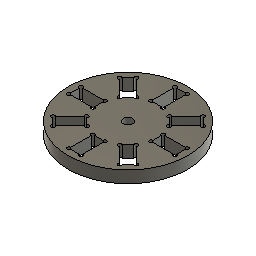
Yatsı Mıknatıs Tutucu v15 (Autodesk Fusion 360 design; units mm, degrees)
Autodesk Fusion 360 part; units mm, degrees
sketch "Eskiz1" plane through (0, 0, 0) normal (0, 1, 0) x (1, 0, 0)
  circle A0 centre (0, 0) radius 20
  circle A1 centre (0, 0) radius 50
  line L0 (-5, 44.3809) -> (5, 44.3809)
  line L1 (5, 44.3809) -> (5, 24.3809)
  line L2 (5, 24.3809) -> (-5, 24.3809)
  line L3 (-5, 24.3809) -> (-5, 44.3809)
  circle A2 centre (-5, 24.3809) radius 1.5
  circle A3 centre (5, 24.3809) radius 1.5
  circle A4 centre (-5, 44.3809) radius 1.5
  circle A5 centre (5, 44.3809) radius 1.5
  circle A6 centre (-34.9176, 27.8465) radius 1.5
  line L4 (-34.9176, 27.8465) -> (-27.8465, 34.9176)
  line L5 (-20.7754, 13.7044) -> (-34.9176, 27.8465)
  line L6 (-13.7044, 20.7754) -> (-20.7754, 13.7044)
  line L7 (-27.8465, 34.9176) -> (-13.7044, 20.7754)
  circle A7 centre (-27.8465, 34.9176) radius 1.5
  circle A8 centre (-20.7754, 13.7044) radius 1.5
  circle A9 centre (-13.7044, 20.7754) radius 1.5
  circle A10 centre (-44.3809, -5) radius 1.5
  line L8 (-44.3809, -5) -> (-44.3809, 5)
  line L9 (-24.3809, -5) -> (-44.3809, -5)
  line L10 (-24.3809, 5) -> (-24.3809, -5)
  line L11 (-44.3809, 5) -> (-24.3809, 5)
  circle A11 centre (-44.3809, 5) radius 1.5
  circle A12 centre (-24.3809, -5) radius 1.5
  circle A13 centre (-24.3809, 5) radius 1.5
  circle A14 centre (-27.8465, -34.9176) radius 1.5
  line L12 (-27.8465, -34.9176) -> (-34.9176, -27.8465)
  line L13 (-13.7044, -20.7754) -> (-27.8465, -34.9176)
  line L14 (-20.7754, -13.7044) -> (-13.7044, -20.7754)
  line L15 (-34.9176, -27.8465) -> (-20.7754, -13.7044)
  circle A15 centre (-34.9176, -27.8465) radius 1.5
  circle A16 centre (-13.7044, -20.7754) radius 1.5
  circle A17 centre (-20.7754, -13.7044) radius 1.5
  circle A18 centre (5, -44.3809) radius 1.5
  line L16 (5, -44.3809) -> (-5, -44.3809)
  line L17 (5, -24.3809) -> (5, -44.3809)
  line L18 (-5, -24.3809) -> (5, -24.3809)
  line L19 (-5, -44.3809) -> (-5, -24.3809)
  circle A19 centre (-5, -44.3809) radius 1.5
  circle A20 centre (5, -24.3809) radius 1.5
  circle A21 centre (-5, -24.3809) radius 1.5
  circle A22 centre (34.9176, -27.8465) radius 1.5
  line L20 (34.9176, -27.8465) -> (27.8465, -34.9176)
  line L21 (20.7754, -13.7044) -> (34.9176, -27.8465)
  line L22 (13.7044, -20.7754) -> (20.7754, -13.7044)
  line L23 (27.8465, -34.9176) -> (13.7044, -20.7754)
  circle A23 centre (27.8465, -34.9176) radius 1.5
  circle A24 centre (20.7754, -13.7044) radius 1.5
  circle A25 centre (13.7044, -20.7754) radius 1.5
  circle A26 centre (44.3809, 5) radius 1.5
  line L24 (44.3809, 5) -> (44.3809, -5)
  line L25 (24.3809, 5) -> (44.3809, 5)
  line L26 (24.3809, -5) -> (24.3809, 5)
  line L27 (44.3809, -5) -> (24.3809, -5)
  circle A27 centre (44.3809, -5) radius 1.5
  circle A28 centre (24.3809, 5) radius 1.5
  circle A29 centre (24.3809, -5) radius 1.5
  circle A30 centre (27.8465, 34.9176) radius 1.5
  line L28 (27.8465, 34.9176) -> (34.9176, 27.8465)
  line L29 (13.7044, 20.7754) -> (27.8465, 34.9176)
  line L30 (20.7754, 13.7044) -> (13.7044, 20.7754)
  line L31 (34.9176, 27.8465) -> (20.7754, 13.7044)
  circle A31 centre (34.9176, 27.8465) radius 1.5
  circle A32 centre (13.7044, 20.7754) radius 1.5
  circle A33 centre (20.7754, 13.7044) radius 1.5
  circle A34 centre (0, 0) radius 3.9
  point P0 (-5, 0)
  point P1 (5, 0)
  dimension "d1" = 40
  dimension "d2" = 100
  dimension "d3" = 5
  dimension "d4" = 5
  dimension "d5" = 10
  dimension "d6" = 20
  dimension "d9" = 44.3809
  dimension "d10" = 3
  dimension "d11" = 3
  dimension "d12" = 3
  dimension "d13" = 3
  dimension "d15" = 360
  dimension "d16" = 7.8
  constraint coincident A0.centre A1.centre
  constraint concentric A0 A1
  constraint horizontal L0
  constraint vertical L1
  constraint horizontal L2
  constraint vertical L3
  constraint coincident L2.end L3.start
  constraint coincident L1.end L2.start
  constraint coincident L0.start L3.end
  constraint coincident L0.end L1.start
  measures "d1" diameter of A0
  measures "d2" diameter of A1
  measures "d3" distance of A0.centre P0
  measures "d4" distance of A0.centre P1
  measures "d5" distance of L0.start L0.end
  measures "d6" distance of L0.start L2.end
  measures "d9" distance of P0 L0.start
  measures "d10" diameter of A2
  measures "d11" diameter of A3
  measures "d12" diameter of A4
  measures "d13" diameter of A5
  measures "d16" diameter of A34
extrude "Ekstrüde Et1" add sketch "Eskiz1" along normal blind 10 contours A0 | A1
extrude "Ekstrüde Et2" add sketch "Eskiz1" along normal blind 6.5 contours A0
sketch "Eskiz2" plane through (0, 10, 0) normal (0, 1, 0) x (-1, 0, 0)
  arc A0 (-14.765, -21.8361) -> (-14.765, -19.7148) centre (-13.7044, -20.7754) ccw
  line L0 (-14.765, -21.8361) -> (-26.7858, -33.8569)
  arc A1 (-28.9072, -33.8569) -> (-26.7858, -33.8569) centre (-27.8465, -34.9176) ccw
  line L1 (-28.9072, -33.8569) -> (-33.8569, -28.9072)
  arc A2 (-33.8569, -26.7858) -> (-33.8569, -28.9072) centre (-34.9176, -27.8465) ccw
  line L2 (-33.8569, -26.7858) -> (-21.8361, -14.765)
  arc A3 (-19.7148, -14.765) -> (-21.8361, -14.765) centre (-20.7754, -13.7044) ccw
  line L3 (-19.7148, -14.765) -> (-14.765, -19.7148)
  circle A4 centre (0, 0) radius 3.9
  arc A5 (-3.5, -24.3809) -> (-5, -25.8809) centre (-5, -24.3809) ccw
  line L4 (-3.5, -24.3809) -> (3.5, -24.3809)
  arc A6 (5, -25.8809) -> (3.5, -24.3809) centre (5, -24.3809) ccw
  line L5 (5, -25.8809) -> (5, -42.8809)
  arc A7 (3.5, -44.3809) -> (5, -42.8809) centre (5, -44.3809) ccw
  line L6 (3.5, -44.3809) -> (-3.5, -44.3809)
  arc A8 (-5, -42.8809) -> (-3.5, -44.3809) centre (-5, -44.3809) ccw
  line L7 (-5, -42.8809) -> (-5, -25.8809)
  arc A9 (21.8361, -14.765) -> (19.7148, -14.765) centre (20.7754, -13.7044) ccw
  line L8 (21.8361, -14.765) -> (33.8569, -26.7858)
  arc A10 (33.8569, -28.9072) -> (33.8569, -26.7858) centre (34.9176, -27.8465) ccw
  line L9 (33.8569, -28.9072) -> (28.9072, -33.8569)
  arc A11 (26.7858, -33.8569) -> (28.9072, -33.8569) centre (27.8465, -34.9176) ccw
  line L10 (26.7858, -33.8569) -> (14.765, -21.8361)
  arc A12 (14.765, -19.7148) -> (14.765, -21.8361) centre (13.7044, -20.7754) ccw
  line L11 (14.765, -19.7148) -> (19.7148, -14.765)
  arc A13 (25.8809, 5) -> (24.3809, 3.5) centre (24.3809, 5) ccw
  line L12 (25.8809, 5) -> (42.8809, 5)
  arc A14 (44.3809, 3.5) -> (42.8809, 5) centre (44.3809, 5) ccw
  line L13 (44.3809, 3.5) -> (44.3809, -3.5)
  arc A15 (42.8809, -5) -> (44.3809, -3.5) centre (44.3809, -5) ccw
  line L14 (42.8809, -5) -> (25.8809, -5)
  arc A16 (24.3809, -3.5) -> (25.8809, -5) centre (24.3809, -5) ccw
  line L15 (24.3809, -3.5) -> (24.3809, 3.5)
  arc A17 (14.765, 21.8361) -> (14.765, 19.7148) centre (13.7044, 20.7754) ccw
  line L16 (14.765, 21.8361) -> (26.7858, 33.8569)
  arc A18 (28.9072, 33.8569) -> (26.7858, 33.8569) centre (27.8465, 34.9176) ccw
  line L17 (28.9072, 33.8569) -> (33.8569, 28.9072)
  arc A19 (33.8569, 26.7858) -> (33.8569, 28.9072) centre (34.9176, 27.8465) ccw
  line L18 (33.8569, 26.7858) -> (21.8361, 14.765)
  arc A20 (19.7148, 14.765) -> (21.8361, 14.765) centre (20.7754, 13.7044) ccw
  line L19 (19.7148, 14.765) -> (14.765, 19.7148)
  arc A21 (-5, 25.8809) -> (-3.5, 24.3809) centre (-5, 24.3809) ccw
  line L20 (-5, 25.8809) -> (-5, 42.8809)
  arc A22 (-3.5, 44.3809) -> (-5, 42.8809) centre (-5, 44.3809) ccw
  line L21 (-3.5, 44.3809) -> (3.5, 44.3809)
  arc A23 (5, 42.8809) -> (3.5, 44.3809) centre (5, 44.3809) ccw
  line L22 (5, 42.8809) -> (5, 25.8809)
  arc A24 (3.5, 24.3809) -> (5, 25.8809) centre (5, 24.3809) ccw
  line L23 (3.5, 24.3809) -> (-3.5, 24.3809)
  arc A25 (-33.8569, 28.9072) -> (-33.8569, 26.7858) centre (-34.9176, 27.8465) ccw
  line L24 (-33.8569, 28.9072) -> (-28.9072, 33.8569)
  arc A26 (-26.7858, 33.8569) -> (-28.9072, 33.8569) centre (-27.8465, 34.9176) ccw
  line L25 (-26.7858, 33.8569) -> (-14.765, 21.8361)
  arc A27 (-14.765, 19.7148) -> (-14.765, 21.8361) centre (-13.7044, 20.7754) ccw
  line L26 (-14.765, 19.7148) -> (-19.7148, 14.765)
  arc A28 (-21.8361, 14.765) -> (-19.7148, 14.765) centre (-20.7754, 13.7044) ccw
  line L27 (-21.8361, 14.765) -> (-33.8569, 26.7858)
  arc A29 (-44.3809, -3.5) -> (-42.8809, -5) centre (-44.3809, -5) ccw
  line L28 (-44.3809, -3.5) -> (-44.3809, 3.5)
  arc A30 (-42.8809, 5) -> (-44.3809, 3.5) centre (-44.3809, 5) ccw
  line L29 (-42.8809, 5) -> (-25.8809, 5)
  arc A31 (-24.3809, 3.5) -> (-25.8809, 5) centre (-24.3809, 5) ccw
  line L30 (-24.3809, 3.5) -> (-24.3809, -3.5)
  arc A32 (-25.8809, -5) -> (-24.3809, -3.5) centre (-24.3809, -5) ccw
  line L31 (-25.8809, -5) -> (-42.8809, -5)
  circle A33 centre (0, 0) radius 50
